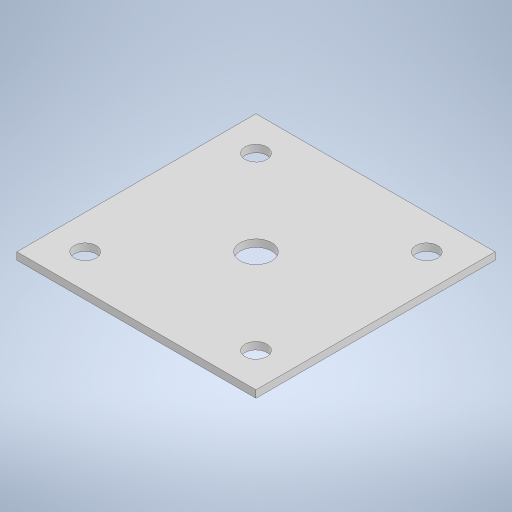
# Autodesk Inventor part: Part3
Saved by Autodesk Inventor 2024.1 (Build 281209000, 209)
## iProperties
Created: 2023-12-23
Part Number: Part3
Material: Generic
Document SubType Name: Modeling
Designer: ryanm
Density: 1 g/cm^3
Appearance: Default
Author: ryanm
Autodesk Inventor part; units mm, degrees
ref_plane "YZ Plane" through (0, 0, 0) normal (1, 0, 0) x (0, 1, 0)
ref_plane "XZ Plane" through (0, 0, 0) normal (0, 1, 0) x (-1, 0, 0)
ref_plane "XY Plane" through (0, 0, 0) normal (0, 0, 1) x (1, 0, 0)
sketch "Sketch1" plane through (0, 0, 0) normal (0, 1, 0) x (-1, 0, 0)
  line L0 (49, -49) -> (-49, -49)
  line L1 (-49, -49) -> (-49, 49)
  line L2 (-49, 49) -> (49, 49)
  line L3 (49, 49) -> (49, -49)
  point P0 (0, 0)
  point P1 (0, -49)
  point P2 (49, 0)
  dimension "d0" = 98
  dimension "d1" = 98
  constraints: 8 end point, 2 midpoint, 2 parallel, 1 horizontal, 1 horizontal alignment, 1 perpendicular, 1 vertical alignment
  measures "d0" distance of L0.start L0.end
  measures "d1" distance of L2.end L0.start
extrude "Extrusion1" add sketch "Sketch1" along normal blind 3
sketch "Sketch2" plane through (0, 3, 0) normal (0, 1, 0) x (1, 0, 0)
  circle A0 centre (0, 0) radius 6.5
  dimension "d4" = 13
  constraints: 1 centre point, 1 coincident
  measures "d4" diameter of A0
extrude "Extrusion2" cut sketch "Sketch2" against normal through all
sketch "Sketch3" plane through (0, 3, 0) normal (0, 1, 0) x (1, 0, 0)
  circle A0 centre (-35, 35) radius 4.5
  circle A1 centre (35, 35) radius 4.5
  circle A2 centre (35, -35) radius 4.5
  circle A3 centre (-35, -35) radius 4.5
  line L0 (49, 49) -> (-49, 49) projected
  line L1 (-49, 49) -> (-49, -49) projected
  line L2 (49, -49) -> (49, 49) projected
  line L3 (-49, -49) -> (49, -49) projected
  point P0 (0, 0)
  dimension "d7" = 9
  dimension "d8" = 9
  dimension "d9" = 9
  dimension "d10" = 9
  dimension "d11" = 14
  dimension "d12" = 14
  dimension "d13" = 14
  dimension "d14" = 14
  constraints: 4 centre point, 2 horizontal alignment, 2 vertical alignment
  measures "d7" diameter of A0
  measures "d8" diameter of A1
  measures "d9" diameter of A2
  measures "d10" diameter of A3
  measures "d11" distance from line of L0 A0.centre
  measures "d12" distance from line of L1 A0.centre
  measures "d13" distance from line of L2 A2.centre
  measures "d14" distance from line of L3 A2.centre
extrude "Extrusion3" cut sketch "Sketch3" against normal through all contours A0 | A1 | A2 | A3
equation "\"d8\" = d7"
equation "\"d9\" = d7"
equation "\"d10\" = d7"
equation "\"d13\" = d12"
equation "\"d14\" = d11"
body "Solid1"
